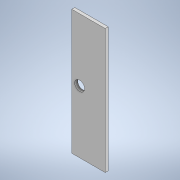
# Autodesk Inventor part: top-1
Saved by Autodesk Inventor 2021 (Build 250183000, 183)
## iProperties
Created: 2024-06-01
Part Number: top-1
Material: Generic
Document SubType Name: Modeling
Designer: user
Density: 1 g/cm^3
Appearance: Default
Author: user
Autodesk Inventor part; units mm, degrees
ref_plane "YZ Plane" through (0, 0, 0) normal (1, 0, 0) x (0, 1, 0)
ref_plane "XZ Plane" through (0, 0, 0) normal (0, 1, 0) x (-1, 0, 0)
ref_plane "XY Plane" through (0, 0, 0) normal (0, 0, 1) x (1, 0, 0)
sketch "Sketch1" plane through (0, 0, 0) normal (0, 0, 1) x (1, 0, 0)
  line L0 (-11, 43) -> (13, 43)
  line L1 (13, 43) -> (13, -43)
  line L2 (13, -43) -> (-11, -43)
  line L3 (-11, -43) -> (-11, 43)
  point P0 (0, 0)
  dimension "d0" = 24
  dimension "d1" = 86
  dimension "d2" = 43
  dimension "d3" = 11
  constraints: 8 end point, 2 parallel, 1 horizontal, 1 perpendicular
  measures "d0" distance of L0.start L0.end
  measures "d1" distance of L0.end L1.end
  measures "d2" distance from line of point (0, 0) L0
  measures "d3" distance from line of point (0, 0) L3
extrude "Extrusion1" add sketch "Sketch1" along normal blind 2
sketch "Sketch2" plane through (0, 0, 2) normal (0, 0, 1) x (1, 0, 0)
  circle A0 centre (-5.8, 0) radius 3.25
  line L0 (13, -43) -> (13, 43) projected
  point P0 (0, 0)
  dimension "d6" = 6.5
  dimension "d7" = 18.8
  constraints: 1 centre point
  measures "d6" diameter of A0
  measures "d7" distance from line of L0 A0.centre
extrude "Extrusion2" cut sketch "Sketch2" against normal blind 2
sketch "Sketch3" plane through (0, 0, 2) normal (0, 0, 1) x (1, 0, 0)
  line L0 (13, 43) -> (-11, 43) projected
  line L1 (13, -43) -> (13, 43) projected
  line L2 (-11, 43) -> (13, 43)
  line L3 (13, 43) -> (13, 41)
  line L4 (13, 41) -> (-11, 41)
  line L5 (-11, 41) -> (-11, 43)
  line L6 (-11, -43) -> (13, -43)
  line L7 (13, -43) -> (13, -41)
  line L8 (13, -41) -> (-11, -41)
  line L9 (-11, -41) -> (-11, -43)
  line L10 (13, -41) -> (11, -41)
  line L11 (11, -41) -> (11, 41)
  line L12 (11, 41) -> (13, 41)
  line L13 (13, 41) -> (13, -41)
  line L14 (-11, 43) -> (-11, -43) projected
  line L15 (-11, -43) -> (13, -43) projected
  point P0 (0, 0)
  dimension "d10" = 2
  dimension "d11" = 2
  dimension "d12" = 2
  constraints: 24 end point, 6 parallel, 3 horizontal, 3 perpendicular, 3 point on line, 2 collinear
  measures "d10" distance between parallel lines of L4 L0
  measures "d11" distance between parallel lines of L1 L11
  measures "d12" distance between parallel lines of L6 L8
extrude "Extrusion3" cut sketch "Sketch3" against normal blind 2 contours L1 L4 L5 L0 | L1 L8 L11 L4 | L1 L6 L9 L8
body "Solid1"
